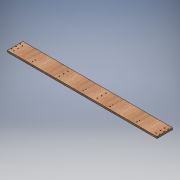
# Autodesk Inventor part: licht_150_front
Saved by Autodesk Inventor 2016 SP2 (Build 200236200, 236)
## iProperties
Created: 2018-01-11
Part Number: licht_150_front
Material: Spanplatte
Document SubType Name: Modeling
Designer: schueler
Density: 1 g/cm^3
Appearance: Birke - natur- poliert
Mass: 3194.24 g
Surface Area: 4575.29 cm^2
Volume: 3194.24 cm^3
Author: schueler
Autodesk Inventor part; units mm, degrees
ref_plane "YZ Plane" through (0, 0, 0) normal (1, 0, 0) x (0, 1, 0)
ref_plane "XZ Plane" through (0, 0, 0) normal (0, 1, 0) x (-1, 0, 0)
ref_plane "XY Plane" through (0, 0, 0) normal (0, 0, 1) x (1, 0, 0)
sketch "Skizze1" plane through (0, 0, 0) normal (0, 0, 1) x (1, 0, 0)
  line L0 (0, 0) -> (1392, 0)
  line L1 (1392, 0) -> (1392, 144)
  line L2 (1392, 144) -> (0, 144)
  line L3 (0, 144) -> (0, 0)
  line L4 (0, 25) -> (1392, 25) construction
  line L5 (0, 50) -> (1392, 50) construction
  line L6 (680, 0) -> (680, 144) construction
  line L7 (930, 144) -> (930, 0) construction
  line L8 (1180, 144) -> (1180, 0) construction
  line L9 (207.5, 144) -> (207.5, 0) construction
  circle A0 centre (207.5, 50) radius 2.5
  circle A1 centre (680, 50) radius 2.5
  circle A2 centre (930, 50) radius 2.5
  circle A3 centre (1180, 50) radius 2.5
  circle A4 centre (1180, 25) radius 3.5
  circle A5 centre (930, 25) radius 3.5
  circle A6 centre (680, 25) radius 3.5
  circle A7 centre (207.5, 25) radius 3.5
  line L10 (1384, 144) -> (1384, 0) construction
  line L11 (1392, 112) -> (0, 112) construction
  line L12 (1392, 32) -> (0, 32) construction
  circle A8 centre (1384, 112) radius 1.5
  circle A9 centre (1384, 32) radius 1.5
  line L13 (8, 144) -> (8, 0) construction
  circle A10 centre (8, 112) radius 1.5
  circle A11 centre (8, 72) radius 1.5
  circle A12 centre (8, 32) radius 1.5
  circle A13 centre (1384, 72) radius 1.5
  circle A14 centre (1359, 25) radius 1.5
  circle A15 centre (1359, 65) radius 1.5
  circle A16 centre (1359, 105) radius 1.5
  circle A17 centre (33, 65) radius 1.5
  line L14 (1359, 25) -> (1359, 105) construction
  line L15 (0, 72) -> (33, 72) construction
  circle A18 centre (33, 105) radius 1.5
  circle A19 centre (33, 25) radius 1.5
  line L16 (33, 25) -> (33, 105) construction
  point P0 (1392, 72)
  dimension "d0" = 1392
  dimension "d1" = 144
  dimension "d2" = 25
  dimension "d3" = 50
  dimension "d6" = 250
  dimension "d8" = 5
  dimension "d9" = 5
  dimension "d10" = 5
  dimension "d11" = 5
  dimension "d12" = 7
  dimension "d13" = 7
  dimension "d14" = 7
  dimension "d15" = 7
  dimension "d20" = 8
  dimension "d21" = 40
  dimension "d22" = 40
  dimension "d23" = 3
  dimension "d24" = 3
  dimension "d25" = 8
  dimension "d26" = 3
  dimension "d27" = 3
  dimension "d28" = 3
  dimension "d29" = 3
  dimension "d137" = 3
  dimension "d138" = 3
  dimension "d139" = 3
  dimension "d143" = 3
  dimension "d153" = 3
  dimension "d154" = 3
  dimension "d206" = 33
  dimension "d210" = 40
  dimension "d211" = 40
  dimension "d212" = 33
  dimension "d213" = 40
  dimension "d214" = 40
  dimension "d215" = 250
  dimension "d216" = 680
  dimension "d217" = 207.5
  constraints: 47 point on line, 34 end point, 20 centre point, 10 perpendicular, 6 midpoint, 3 coincident, 3 parallel, 2 horizontal, 2 vertical
  measures "d0" distance of L2.end L1.end
  measures "d1" distance of L1.end L0.end
  measures "d2" distance of L0.end L4.end
  measures "d3" distance of L0.end L5.end
  measures "d6" distance of L8.start L7.start
  measures "d8" diameter of A0
  measures "d9" diameter of A1
  measures "d10" diameter of A2
  measures "d11" diameter of A3
  measures "d12" diameter of A4
  measures "d13" diameter of A5
  measures "d14" diameter of A6
  measures "d15" diameter of A7
  measures "d20" distance of L1.end L10.start
  measures "d21" distance of L11.start point (1392, 72)
  measures "d22" distance of L12.start point (1392, 72)
  measures "d23" diameter of A8
  measures "d24" diameter of A9
  measures "d25" distance of L13.start L2.end
  measures "d26" diameter of A10
  measures "d27" diameter of A11
  measures "d28" diameter of A12
  measures "d29" diameter of A13
  measures "d137" diameter of A14
  measures "d138" diameter of A15
  measures "d139" diameter of A16
  measures "d143" diameter of A17
  measures "d153" diameter of A18
  measures "d154" diameter of A19
  measures "d206" distance between parallel lines of L3 L16
  measures "d210" distance from line of A17.centre L4
  measures "d211" distance of A17.centre A18.centre
  measures "d212" distance between parallel lines of L1 L14
  measures "d213" distance from line of L4 A15.centre
  measures "d214" distance of A15.centre L14.end
  measures "d215" distance between parallel lines of L7 L6
  measures "d216" distance between parallel lines of L3 L6
  measures "d217" distance between parallel lines of L3 L9
extrude "Extrusion1" add sketch "Skizze1" along normal blind 16
hole "Bohrung1" at (1180, 25, 0) at (930, 25, 0) at (680, 25, 0) at (207.5, 25, 0) direction (0, 0, 1) diameter 10 depth 12 tip angle 118
hole "Bohrung4" at (930, 50, 0) at (680, 50, 0) at (207.5, 50, 0) at (1180, 50, 0) direction (0, 0, 1) diameter 7 depth 12 tip angle 118
sketch "Skizze4" plane through (0, 0, 16) normal (0, 0, 1) x (1, 0, 0)
  circle A0 centre (8, 112) radius 1.5 projected
  circle A1 centre (8, 72) radius 1.5 projected
  circle A2 centre (8, 32) radius 1.5 projected
  circle A3 centre (30, 72) radius 1.5 projected
  circle A4 centre (207.5, 25) radius 3.5 projected
  circle A5 centre (680, 25) radius 3.5 projected
  circle A6 centre (930, 25) radius 3.5 projected
  circle A7 centre (1180, 25) radius 3.5 projected
  circle A8 centre (1180, 50) radius 2.5 projected
  circle A9 centre (930, 50) radius 2.5 projected
  circle A10 centre (680, 50) radius 2.5 projected
  circle A11 centre (207.5, 50) radius 2.5 projected
  circle A12 centre (33, 25) radius 1.5 projected
  circle A13 centre (33, 105) radius 1.5 projected
  circle A14 centre (33, 65) radius 1.5 projected
  circle A15 centre (1359, 105) radius 1.5 projected
  circle A16 centre (1359, 65) radius 1.5 projected
  circle A17 centre (1359, 25) radius 1.5 projected
  circle A18 centre (1384, 72) radius 1.5 projected
  circle A19 centre (8, 32) radius 1.5 projected
  circle A20 centre (8, 72) radius 1.5 projected
  circle A21 centre (8, 112) radius 1.5 projected
  circle A22 centre (1384, 32) radius 1.5 projected
  circle A23 centre (1384, 112) radius 1.5 projected
  line L0 (0, 0) -> (1392, 0) projected
  line L1 (1392, 0) -> (1392, 144) projected
  line L2 (1392, 144) -> (0, 144) projected
  line L3 (0, 144) -> (0, 0) projected
hole "Bohrung15" at (1359, 65, 16) at (1384, 32, 16) at (1384, 72, 16) at (1384, 112, 16) at (1359, 105, 16) at (1359, 25, 16) at (33, 65, 16) at (33, 25, 16) at (33, 105, 16) at (8, 72, 16) at (8, 112, 16) at (8, 32, 16) direction (0, 0, -1) diameter 3 depth 8 tip angle 118 countersink diameter 8 countersink angle 90
sketch "Skizze5" plane through (0, 144, 0) normal (0, 1, 0) x (1, 0, 0)
  line L0 (1392, -16) -> (0, -16) construction
  line L1 (0, -16) -> (0, 0) construction
  line L2 (0, 0) -> (1392, 0) construction
  line L3 (1392, 0) -> (1392, -16) construction
  line L4 (0, 0) -> (0, -16) construction
  line L5 (0, -8) -> (1392, -8) construction
  line L6 (1392, 0) -> (1392, -16) construction
  line L7 (0, -16) -> (1392, -16) construction
  line L8 (696, -16) -> (696, 0) construction
  line L9 (0, 0) -> (1392, 0) construction
  point P0 (0, 0)
  point P1 (700, -8)
  point P2 (900, -8)
  point P3 (1100, -8)
  point P4 (1300, -8)
  point P5 (500, -8)
  point P6 (300, -8)
  point P7 (100, -8)
  dimension "d190" = 200
  dimension "d191" = 200
  dimension "d195" = 200
  dimension "d196" = 200
  dimension "d197" = 200
  dimension "d244" = 200
  dimension "d245" = 100
  dimension "d246" = 92
  constraints: 10 end point, 4 midpoint, 2 parallel, 1 horizontal, 1 perpendicular, 10 other
  measures "d190" distance of point (300, -8) point (500, -8)
  measures "d191" distance of point (100, -8) point (300, -8)
  measures "d195" distance of point (700, -8) point (900, -8)
  measures "d196" distance of point (900, -8) point (1100, -8)
  measures "d197" distance of point (1100, -8) point (1300, -8)
  measures "d244" distance of point (500, -8) point (700, -8)
  measures "d245" distance from line of L1 point (100, -8)
  measures "d246" distance from line of point (1300, -8) L3
hole "Bohrung16" at (1300, 144, 8) at (1100, 144, 8) at (900, 144, 8) at (500, 144, 8) at (300, 144, 8) at (100, 144, 8) at (700, 144, 8) direction (0, -1, 0) diameter 3 depth 30 tip angle 118
sketch "Skizze7" plane through (0, 0, 16) normal (0, 0, 1) x (1, 0, 0)
  line L0 (1392, 144) -> (0, 144) construction
  line L1 (0, 0) -> (1392, 0) construction
  line L2 (0, 144) -> (0, 0) construction
  line L3 (1392, 0) -> (1392, 144) construction
  line L4 (450, 0) -> (450, 144) construction
  line L5 (805, 0) -> (805, 144) construction
  circle A0 centre (680, 50) radius 2.5 construction
  line L6 (450, 32) -> (805, 32) construction
  line L7 (805, 112) -> (450, 112) construction
  point P0 (450, 72)
  point P1 (805, 72)
  dimension "d226" = 450
  dimension "d227" = 125
  dimension "d228" = 40
  dimension "d229" = 40
  constraints: 8 end point, 8 point on line, 2 midpoint, 2 perpendicular, 1 horizontal, 1 parallel
  measures "d226" distance between parallel lines of L4 L2
  measures "d227" distance from line of A0.centre L5
  measures "d228" distance from line of L7 point (805, 72)
  measures "d229" distance of point (805, 72) L6.end
hole "Bohrung17" at (805, 32, 16) at (805, 72, 16) at (805, 112, 16) direction (0, 0, -1) diameter 3 end through all countersink diameter 8 countersink angle 90
hole "Bohrung18" at (450, 72, 16) at (450, 112, 16) at (450, 32, 16) direction (0, 0, -1) diameter 8 end through all
